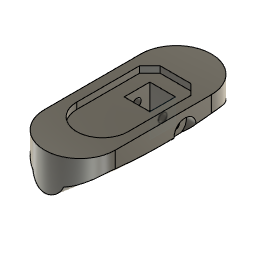
ClimbSim_FootPart v6 (Autodesk Fusion 360 design; units mm, degrees)
Autodesk Fusion 360 part; units mm, degrees
sketch "スケッチ2" plane through (0, 0, 0) normal (0, 0, 1) x (1, 0, 0)
  line L0 (27.5, 37.5) -> (27.5, -37.5)
  line L1 (-27.5, -37.5) -> (-27.5, 37.5)
  arc A0 (27.5, 37.5) -> (-27.5, 37.5) centre (0, 37.5) ccw
  arc A1 (-27.5, -37.5) -> (27.5, -37.5) centre (0, -37.5) ccw
  dimension "d2" = 27.5
  dimension "d3" = 75
  dimension "d4" = 37.5
  constraint vertical L0
  constraint vertical L1
  constraint coincident L0.start A0.start
  constraint tangent L1 A1
  constraint tangent L1 A0
  constraint tangent L0 A1
  constraint tangent L0 A0
  constraint vertical origin A0.centre
  measures "d2" radius of A0
  measures "d3" distance of L0.start L0.end
  measures "d4" distance of origin A0.centre
extrude "押し出し1" add sketch "スケッチ2" along normal blind 50
sketch "スケッチ3" plane through (0, 0, 50) normal (0, 0, 1) x (-1, 0, 0)
  arc A0 (-27.5, -37.5) -> (27.5, -37.5) centre (0, -37.5) ccw
  line L0 (27.5, -37.5) -> (27.5, 37.5)
  arc A1 (27.5, 37.5) -> (-27.5, 37.5) centre (0, 37.5) ccw
  line L1 (-27.5, 37.5) -> (-27.5, -37.5)
  line L2 (20, -29) -> (20, 20)
  arc A2 (20, 20) -> (-20, 20) centre (0, 20) ccw
  line L3 (-20, 20) -> (-20, -29)
  line L4 (-20, -29) -> (-12, -37)
  line L5 (-12, -37) -> (12, -37)
  line L6 (12, -37) -> (20, -29)
  dimension "d7" = 20
  dimension "d8" = 57
  dimension "d9" = 24
  dimension "d45" = 20
  constraint vertical L2
  constraint parallel L0 L3
  constraint perpendicular L3 L5
  constraint tangent A2 L3
  constraint horizontal L2.start L3.end
  constraint tangent L2 A2
  constraint equal L4 L6
  constraint perpendicular L4 L6
  constraint vertical origin A2.centre
  measures "d7" radius of A2
  measures "d8" vertical distance of A2.centre L5.end
  measures "d9" distance of L4.end L5.end
  measures "d45" distance of origin A2.centre
extrude "押し出し2" cut sketch "スケッチ3" against normal blind 20 contours L2 A2 L3 L4 L5 L6
sketch "スケッチ4" plane through (0, 0, 30) normal (0, 0, 1) x (-1, 0, 0)
  line L0 (12, -37) -> (20, -29)
  line L1 (20, -29) -> (20, 20)
  arc A0 (20, 20) -> (-20, 20) centre (0, 20) ccw
  line L2 (-20, 20) -> (-20, -29)
  line L3 (-20, -29) -> (-12, -37)
  line L4 (-12, -37) -> (12, -37)
  line L5 (10, -27) -> (-10, -27)
  line L6 (-10, -27) -> (-10, -7)
  line L7 (-10, -7) -> (10, -7)
  line L8 (10, -7) -> (10, -27)
  dimension "d14" = 10
  dimension "d48" = 10
  dimension "d49" = 10
  constraint horizontal L5
  constraint vertical L6
  constraint horizontal L7
  constraint vertical L8
  constraint equal L7 L8
  measures "d14" vertical distance of L0.start L5.start
  measures "d48" distance of L1 L7.end
  measures "d49" distance of L2 L6.end
extrude "押し出し3" cut sketch "スケッチ4" against normal blind 19 contours L5 L6 L7 L8
sketch "スケッチ5" plane through (0, 0, 0) normal (0, 1, 0) x (1, 0, 0)
  arc A0 (12, -9) -> (-12, -9) centre (0, -12.5) ccw
  line L0 (35, -41.8786) -> (35, 32.3347)
  line L1 (35, 32.3347) -> (-35, 32.3347)
  line L2 (-35, 32.3347) -> (-35, -41.8786)
  line L3 (75, -350) -> (-75, -350)
  line L4 (-27.5, 0) -> (27.5, 0)
  arc A1 (35, -41.8786) -> (12, -9) centre (0, -41.8786) ccw
  arc A2 (-12, -9) -> (-35, -41.8786) centre (0, -41.8786) ccw
  dimension "d18" = 12.5
  dimension "d19" = 350
  dimension "d23" = 70
  dimension "d24" = 35
  constraint perpendicular L0 L1
  constraint perpendicular L1 L2
  constraint vertical origin A0.centre
  constraint horizontal L3
  constraint tangent A0 L4
  constraint vertical L0
  constraint horizontal L0.start L2.end
  constraint horizontal A0.start A0.end
  constraint coincident L0.start A1.start
  constraint equal A1 A2
  constraint coincident A1.centre A2.centre
  measures "d18" radius of A0
  measures "d19" vertical distance of origin L3.start
  measures "d23" distance of L0.end L1.end
  measures "d24" radius of A1
revolve "回転1" cut sketch "スケッチ5" angle 360 about axis through (75, 0, 350) along (-1, 0, 0)
sketch "スケッチ9" plane through (10, 0, 0) normal (-1, 0, 0) x (0, -1, 0)
  line L0 (-7, 30) -> (-27, 30)
  line L1 (-27, 30) -> (-27, 11)
  line L2 (-27, 11) -> (-7, 11)
  line L3 (-7, 11) -> (-7, 30)
  circle A0 centre (-17, 21) radius 3.25
  dimension "d31" = 6.5
  dimension "d32" = 9
  dimension "d33" = 10
  measures "d31" diameter of A0
  measures "d32" distance of L0 A0.centre
  measures "d33" distance of L3 A0.centre
extrude "押し出し6" cut sketch "スケッチ9" along normal through all and the other way through all contours A0
sketch "スケッチ14" plane through (0, 0, 0) normal (1, 0, 0) x (0, 1, 0)
  circle A0 centre (17, 21) radius 8.544
  point P0 (17, 21)
  dimension "d40" = 17.088
  constraint coincident P0 A0.centre
  measures "d40" diameter of A0
extrude "押し出し8" cut sketch "スケッチ14" along normal blind 20 from surface at 20
mirror "ミラー1" about plane through (0, 0, 0) normal (1, 0, 0) of "押し出し8"
sketch "スケッチ15" plane through (0, 0, 50) normal (0, 0, 1) x (-1, 0, 0)
  line L0 (20, 20) -> (20, -29)
  line L1 (20, -29) -> (12, -37)
  line L2 (12, -37) -> (-12, -37)
  line L3 (-12, -37) -> (-20, -29)
  line L4 (-20, -29) -> (-20, 20)
  arc A0 (20, 20) -> (-20, 20) centre (0, 20) ccw
  arc A1 (-27.5, -37.5) -> (27.5, -37.5) centre (0, -37.5) ccw
  line L5 (27.5, -37.5) -> (27.5, 37.5)
  arc A2 (27.5, 37.5) -> (-27.5, 37.5) centre (0, 37.5) ccw
  line L6 (-27.5, 37.5) -> (-27.5, -37.5)
  line L7 (42.7311, -72.162) -> (-49.8708, -72.162)
  line L8 (-49.8708, -72.162) -> (-49.8708, 74.8211)
  line L9 (-49.8708, 74.8211) -> (42.7311, 74.8211)
  line L10 (42.7311, 74.8211) -> (42.7311, -72.162)
  constraint horizontal L7
  constraint vertical L8
  constraint horizontal L9
  constraint vertical L10
extrude "押し出し9" cut sketch "スケッチ15" against normal blind 15 contours A1 L5 A2 L6
